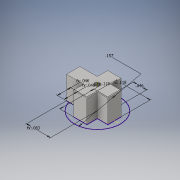
# Autodesk Inventor part: shuttle
Saved by Autodesk Inventor 2016 (Build 200138000, 138)
## iProperties
Created: 2016-07-02
Part Number: shuttle
Material: Generic
Document SubType Name: Modeling
Designer: GentnerLab
Density: 1 g/cm^3
Appearance: Default
Author: GentnerLab
Autodesk Inventor part; units mm, degrees
ref_plane "YZ Plane" through (0, 0, 0) normal (1, 0, 0) x (0, 1, 0)
ref_plane "XZ Plane" through (0, 0, 0) normal (0, 1, 0) x (-1, 0, 0)
ref_plane "XY Plane" through (0, 0, 0) normal (0, 0, 1) x (1, 0, 0)
sketch "base+body" plane through (0, 0, 0) normal (0, 1, 0) x (-1, 0, 0)
  circle A0 centre (0, 0) radius 2
  line L0 (-0.5875, 1.5) -> (0.5875, 1.5)
  line L1 (0.5875, 1.5) -> (0.5875, -1.5)
  line L2 (0.5875, -1.5) -> (-0.5875, -1.5)
  line L3 (-0.5875, -1.5) -> (-0.5875, 1.5)
  line L4 (-0.5875, 1.5) -> (0.5875, -1.5) construction
  line L5 (0.5875, 1.5) -> (-0.5875, -1.5) construction
  line L6 (-1.5, 0.5875) -> (1.5, 0.5875)
  line L7 (1.5, 0.5875) -> (1.5, -0.5875)
  line L8 (1.5, -0.5875) -> (-1.5, -0.5875)
  line L9 (-1.5, -0.5875) -> (-1.5, 0.5875)
  line L10 (-1.5, 0.5875) -> (1.5, -0.5875) construction
  line L11 (1.5, 0.5875) -> (-1.5, -0.5875) construction
  line L12 (0, 0.5875) -> (2.1, 0.5875)
  line L13 (2.1, 0.5875) -> (2.1, -0.5875)
  line L14 (2.1, -0.5875) -> (0, -0.5875)
  line L15 (0, -0.5875) -> (0, 0.5875)
  dimension "d0" = 4
  dimension "d1" = 3
  dimension "d2" = 1.175
  dimension "d3" = 1.175
  dimension "d4" = 3
  dimension "d5" = 1.175
  dimension "d6" = 2.1
  constraints: 32 end point, 6 parallel, 5 midpoint, 3 horizontal, 3 perpendicular, 2 coincident, 1 centre point
  measures "d0" diameter of A0
  measures "d1" distance between parallel lines of L0 L2
  measures "d2" distance between parallel lines of L3 L1
  measures "d3" distance between parallel lines of L8 L6
  measures "d4" distance between parallel lines of L9 L7
  measures "d5" distance between parallel lines of L14 L12
  measures "d6" distance from line of A0.centre L13
extrude "Extrusion6" add sketch "base+body" along normal blind 2 contours A0 L14 L7 L12 | A0 L12 L13 L14 | L7 L8 L1 L6 | L6 L3 L0 L1 | L1 L8 L15 L6 | L1 L2 L3 L8 | L15 L8 L3 L6 | L3 L8 L9 L6
hole "Hole4" at (0, 0, 0) direction (0, 1, 0) diameter 0.45 end through all
equation "\"d3\" = d2"
equation "\"d4\" = d1"
equation "\"d5\" = d2"
body "Solid4"
